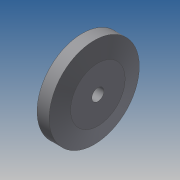
# Autodesk Inventor part: Propellerscheibe_ra8846s
Saved by Autodesk Inventor 2021 (Build 250183000, 183)
## iProperties
Created: 2020-11-16
Part Number: Propellerscheibe_ra8846s
Material: Allgemein
Document SubType Name: Modeling
Designer: Sander
Density: 1 g/cm^3
Appearance: Vorgabe
Author: Sander
Autodesk Inventor part; units mm, degrees
ref_plane "YZ-Ebene" through (0, 0, 0) normal (1, 0, 0) x (0, 1, 0)
ref_plane "XZ-Ebene" through (0, 0, 0) normal (0, 1, 0) x (-1, 0, 0)
ref_plane "XY-Ebene" through (0, 0, 0) normal (0, 0, 1) x (1, 0, 0)
sketch "Skizze1" plane through (0, 0, 0) normal (0, 0, 1) x (1, 0, 0)
  line L0 (-0.5199, 0) -> (3.1196, 0) projected
  line L1 (0, -1.4879) -> (0, 8.9274) projected
  line L2 (0, 7.4395) -> (2, 7.4395)
  line L3 (2, 7.4395) -> (2.5996, 4.5)
  line L4 (2.5996, 4.5) -> (2.5996, 1)
  line L5 (2.5996, 1) -> (0, 1)
  point P0 (0, 0)
  dimension "d2" = 2
  dimension "d3" = 3
  dimension "d4" = 101.53
  dimension "d5" = 3.5
  dimension "d6" = 1
  constraints: 8 end point, 3 perpendicular, 2 point on line
  measures "d2" distance of L2.start L2.end
  measures "d3" distance of L2.end L3.end
  measures "d4" angle of L2 L3
  measures "d5" distance of L3.end L4.end
  measures "d6" distance between parallel lines of L5 L0
revolve "Umdrehung1" add sketch "Skizze1" angle 360 about axis through (-10, 0, 0) along (1, 0, 0)
